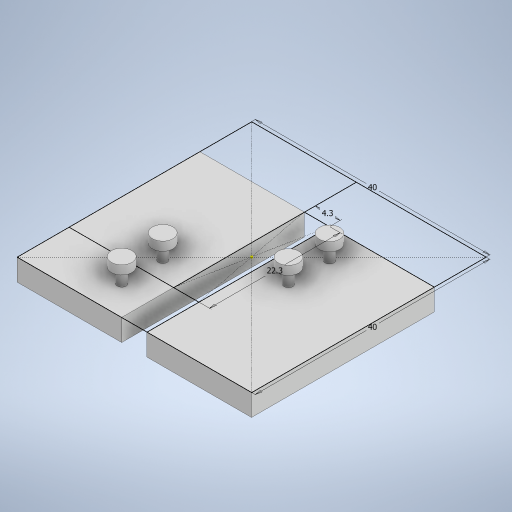
# Autodesk Inventor part: top-big
Saved by Autodesk Inventor 2023 (Build 270158000, 158)
## iProperties
Created: 2023-08-09
Part Number: top-big
Material: Generic
Document SubType Name: Modeling
Designer: AxLab
Density: 1 g/cm^3
Appearance: Default
Author: AxLab
Autodesk Inventor part; units mm, degrees
ref_plane "YZ Plane" through (0, 0, 0) normal (1, 0, 0) x (0, 1, 0)
ref_plane "XZ Plane" through (0, 0, 0) normal (0, 1, 0) x (-1, 0, 0)
ref_plane "XY Plane" through (0, 0, 0) normal (0, 0, 1) x (1, 0, 0)
sketch "Sketch4" plane through (0, 0, 0) normal (0, 1, 0) x (-1, 0, 0)
  line L0 (20, 20) -> (-20, 20)
  line L1 (-20, 20) -> (-20, -20)
  line L2 (-20, -20) -> (20, -20)
  line L3 (20, -20) -> (20, 20)
  line L4 (20, 20) -> (-20, -20) construction
  line L5 (-20, 20) -> (20, -20) construction
  line L6 (2.15, 11.15) -> (-2.15, 11.15)
  line L7 (-2.15, 11.15) -> (-2.15, -11.15)
  line L8 (-2.15, -11.15) -> (2.15, -11.15)
  line L9 (2.15, -11.15) -> (2.15, 11.15)
  line L10 (2.15, 11.15) -> (-2.15, -11.15) construction
  line L11 (-2.15, 11.15) -> (2.15, -11.15) construction
  line L12 (2.15, 11.15) -> (20, 11.15)
  line L13 (20, 11.15) -> (20, -20)
  line L14 (20, -20) -> (2.15, -20)
  line L15 (2.15, -20) -> (2.15, 11.15)
  line L16 (-2.15, -11.15) -> (-20, -11.15)
  line L17 (-20, -11.15) -> (-20, 20)
  line L18 (-20, 20) -> (-2.15, 20)
  line L19 (-2.15, 20) -> (-2.15, -11.15)
  point P0 (0, 0)
  point P1 (-2.15, 20)
  point P2 (2.15, -20)
  dimension "d26" = 40
  dimension "d27" = 40
  dimension "d28" = 4.3
  dimension "d29" = 22.3
  constraints: 40 end point, 8 parallel, 4 horizontal, 4 midpoint, 4 perpendicular
  measures "d26" distance of L2.end L1.end
  measures "d27" distance of L1.end L0.end
  measures "d28" distance of L8.end L7.end
  measures "d29" distance of L7.end L6.end
extrude "Extrusion4" add sketch "Sketch4" along normal blind 3.7 contours L19 L7 L16 L1 L0 | L3 L2 L15 L9 L12
sketch "Sketch5" plane through (0, 0, 0) normal (0, 1, 0) x (-1, 0, 0)
  line L0 (2.15, -20) -> (20, -20) projected
  line L1 (2.15, -20) -> (7.15, -20)
  line L2 (7.15, -20) -> (7.15, -15)
  line L3 (7.15, -15) -> (2.15, -15)
  line L4 (2.15, -15) -> (2.15, -20)
  line L5 (2.15, -20) -> (7.15, -20)
  line L6 (7.15, -20) -> (7.15, -8)
  line L7 (7.15, -8) -> (2.15, -8)
  line L8 (2.15, -8) -> (2.15, -20)
  line L9 (-2.15, -11.15) -> (-2.15, 20) projected
  line L10 (-2.15, 20) -> (-7.15, 20)
  line L11 (-7.15, 20) -> (-7.15, 15)
  line L12 (-7.15, 15) -> (-2.15, 15)
  line L13 (-2.15, 15) -> (-2.15, 20)
  line L14 (-2.15, 20) -> (-7.15, 20)
  line L15 (-7.15, 20) -> (-7.15, 8)
  line L16 (-7.15, 8) -> (-2.15, 8)
  line L17 (-2.15, 8) -> (-2.15, 20)
  circle A0 centre (-7.15, 8) radius 0.75
  circle A1 centre (-7.15, 15) radius 0.75
  circle A2 centre (7.15, -15) radius 0.75
  circle A3 centre (7.15, -8) radius 0.75
  point P0 (0, 0)
  dimension "d32" = 5
  dimension "d33" = 5
  dimension "d34" = 12
  dimension "d35" = 5
  dimension "d36" = 5
  dimension "d37" = 12
  dimension "d38" = 1.5
  dimension "d39" = 1.5
  dimension "d40" = 1.5
  dimension "d41" = 1.5
  constraints: 32 end point, 8 parallel, 4 centre point, 4 coincident, 4 horizontal, 4 perpendicular, 2 point on line
  measures "d32" distance of L3.end L2.end
  measures "d33" distance of L2.end L1.end
  measures "d34" distance of L6.end L5.end
  measures "d35" distance of L12.end L11.end
  measures "d36" distance of L11.end L10.end
  measures "d37" distance of L15.end L14.end
  measures "d38" diameter of A0
  measures "d39" diameter of A1
  measures "d40" diameter of A2
  measures "d41" diameter of A3
extrude "Extrusion5" add sketch "Sketch5" against normal blind 2.5 contours A2 L3 L2 | L2 L6 A2 | A2 L6 L3 | A3 L6 L7 | L7 L6 A3 | A0 L15 L16 | L16 L15 A0 | A1 L15 L12 | L12 L11 A1 | L15 A1 L11
sketch "Sketch6" plane through (-7.15, -2.5, -15) normal (0, -1, 0) x (1, 0, 0)
  circle A0 centre (0, 0) radius 1.75
  circle A1 centre (0, 7) radius 0.75 projected
  circle A2 centre (0, 7) radius 1.75
  circle A3 centre (14.3, 23) radius 0.75 projected
  circle A4 centre (14.3, 23) radius 1.75
  circle A5 centre (14.3, 30) radius 0.75 projected
  circle A6 centre (14.3, 30) radius 1.75
  point P0 (7.15, 15)
  dimension "d44" = 3.5
  dimension "d45" = 3.5
  dimension "d46" = 3.5
  dimension "d47" = 3.5
  constraints: 4 centre point, 3 coincident
  measures "d44" diameter of A0
  measures "d45" diameter of A2
  measures "d46" diameter of A4
  measures "d47" diameter of A6
extrude "Extrusion6" add sketch "Sketch6" along normal blind 1.5 contours A0 | A1 | A2 | A3 | A4 | A5 | A6
move or copy body "Move Body1" bodies to move or copy 1 copy no rotation origin (0, 0, 0) rotation axis (0, 0, 1) rotation angle -180
split body "Split1" sketch "Sketch4" result two bodies curves L18 L19 first body at (-14.05, -3.2, 9.6167)
move or copy body "Move Body2" bodies to move or copy 3 copy no translate (0, 0, 8.85)
body "Solid3"
body "Solid4"
